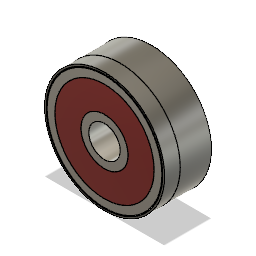
_ball bearing.1ca2f9a9-7553-43a8-93c9-ccd7098722b7 (Autodesk Fusion 360 design; units mm, degrees)
Autodesk Fusion 360 part; units mm, degrees
sketch "Sketch1" plane through (0, 0, 0) normal (0, 0, 1) x (1, 0, 0)
  circle A0 centre (0, 0) radius 3
  circle A1 centre (0, 0) radius 4.5
  circle A2 centre (0, 0) radius 9.5
  circle A3 centre (0, 0) radius 11
  dimension "d1" = 6
  dimension "d2" = 9
  dimension "d3" = 19
  dimension "d4" = 22
  measures "d1" diameter of A0
  measures "d2" diameter of A1
  measures "d3" diameter of A2
  measures "d4" diameter of A3
extrude "Extrude1" add sketch "Sketch1" along normal blind 6 contours A3 makes body 1
extrude "Extrude2" add sketch "Sketch1" along normal blind 6 separate body contours A2 makes body 2
extrude "Extrude3" add sketch "Sketch1" along normal blind 6 separate body contours A1 makes body 3
sketch "Sketch2" plane through (0, 0, 6) normal (0, 0, 1) x (1, 0, 0)
  circle A0 centre (0, 0) radius 9.5
  circle A1 centre (0, 0) radius 11
  circle A2 centre (0, 0) radius 11.5
  circle A3 centre (0, 0) radius 11.15
  dimension "d11" = 22.3
  measures "d11" diameter of A3
extrude "Extrude4" add sketch "Sketch2" against normal blind 3 separate body contours A2 makes body 4
ref_plane "WorkPlane1" through (0, 0, 3) normal (0, 0, 1) x (1, 0, 0)
mirror "Mirror1" about plane through (0, 0, 3) normal (0, 0, 1) of "Extrude4" makes body 5
sketch "Sketch3" plane through (0, 0, 0) normal (0, 0, -1) x (-1, 0, 0)
  circle A0 centre (0, 0) radius 11.15
  circle A1 centre (0, 0) radius 11.5
  circle A2 centre (0, 0) radius 11.5
extrude "Extrude5" add sketch "Sketch3" along normal blind 3 separate body contours A0 | A1 A2 makes body 6
combine "Combine1" operation add target body 5 tool bodies 6
sketch "Sketch4" plane through (0, 0, 6) normal (0, 0, 1) x (1, 0, 0)
  circle A0 centre (0, 0) radius 11.15
  circle A1 centre (0, 0) radius 11.5
  line L0 (-4.9572, 10.4939) -> (-5.6603, 11.5434)
  arc A2 (-5.6603, 11.5434) -> (-8.3245, 9.76) centre (-7.015, 10.6854) ccw
  line L1 (-7.588, 8.7179) -> (-8.3245, 9.76)
  arc A3 (-4.9572, 10.4939) -> (-7.616, 8.7574) centre (0, 0) ccw
